Autodesk Fusion 360 part; units mm, degrees
note: some values were not read from the file. Chosen so that the rebuilt part matches the saved one: which bodies a step acts on; that a step has no effect.
(part 2 of 2)
sketch "Sketch27" plane through (0, 1.55, 0) normal (0, 1, 0) x (-1, 0, 0)
  circle A0 centre (-8.4, -28.1) radius 0.5
  circle A1 centre (-13.4, -28.1) radius 0.5
  circle A2 centre (-18.4, -28.1) radius 0.5
  line L0 (-19.48, -2.52) -> (-19.98, -2.52)
  line L1 (-19.98, -2.52) -> (-19.98, -2.02)
  line L2 (-19.98, -2.02) -> (-19.48, -2.02)
  line L3 (-19.48, -2.02) -> (-19.48, -2.52)
  line L4 (-16.94, -2.52) -> (-17.44, -2.52)
  line L5 (-17.44, -2.52) -> (-17.44, -2.02)
  line L6 (-17.44, -2.02) -> (-16.94, -2.02)
  line L7 (-16.94, -2.02) -> (-16.94, -2.52)
  line L8 (-14.4, -2.52) -> (-14.9, -2.52)
  line L9 (-14.9, -2.52) -> (-14.9, -2.02)
  line L10 (-14.9, -2.02) -> (-14.4, -2.02)
  line L11 (-14.4, -2.02) -> (-14.4, -2.52)
  circle A3 centre (-2.275, -2.375) radius 1.475
  circle A4 centre (-23.725, -2.375) radius 1.475
  circle A5 centre (-23.725, -31.325) radius 1.475
  circle A6 centre (-2.275, -31.325) radius 1.475
  line L12 (0, -33.5) -> (0, 0)
  line L13 (0, 0) -> (-26, 0)
  line L14 (-26, 0) -> (-26, -33.5)
  line L15 (-26, -33.5) -> (0, -33.5)
  circle A7 centre (-2.275, -31.325) radius 1.525
  circle A8 centre (-2.275, -31.325) radius 1.625
  line L16 (-13, -33.5) -> (-13, -31.8167) construction
  circle A9 centre (-23.725, -31.325) radius 1.475
  circle A10 centre (-23.725, -31.325) radius 1.625
  circle A11 centre (-2.275, -2.375) radius 1.525
  circle A12 centre (-2.275, -2.375) radius 1.625
  circle A13 centre (-23.725, -2.375) radius 1.625
  circle A14 centre (-23.725, -2.375) radius 1.525
  line L17 (-13.33, -3.59) -> (-21.05, -3.59)
  line L18 (-21.05, -3.59) -> (-21.05, -0.95)
  line L19 (-21.05, -0.95) -> (-13.33, -0.95)
  line L20 (-13.33, -0.95) -> (-13.33, -3.59)
  line L21 (-13.38, -3.032) -> (-13.38, -1.508)
  line L22 (-15.412, -3.54) -> (-13.888, -3.54)
  line L23 (-18.968, -1) -> (-20.492, -1)
  line L24 (-21, -1.508) -> (-21, -3.032)
  line L25 (-21.15, -0.85) -> (-13.23, -0.85)
  line L26 (-13.23, -0.85) -> (-13.23, -3.69)
  line L27 (-13.23, -3.69) -> (-21.15, -3.69)
  line L28 (-21.15, -3.69) -> (-21.15, -0.85)
  line L29 (-12.6, -0.3) -> (-21.5, -0.3) construction
  line L30 (-7.1042, -0.3) -> (-11.1042, -0.3) construction
  line L31 (-2.45, -19.55) -> (-4.55, -19.55)
  line L32 (-4.55, -19.55) -> (-4.55, -15.05)
  line L33 (-4.55, -15.05) -> (-2.45, -15.05)
  line L34 (-2.45, -15.05) -> (-2.45, -19.55)
  line L35 (-2.5, -19.3) -> (-2.5, -15.3)
  line L36 (-4, -19.5) -> (-3, -19.5)
  line L37 (-4, -15.1) -> (-3, -15.1)
  line L38 (-4.5, -15.3) -> (-4.5, -19.3)
  line L39 (-4.65, -19.65) -> (-4.65, -14.95)
  line L40 (-4.65, -14.95) -> (-2.35, -14.95)
  line L41 (-2.35, -14.95) -> (-2.35, -19.65)
  line L42 (-2.35, -19.65) -> (-4.65, -19.65)
  line L43 (-2.35, -19.65) -> (0, -19.65) construction
  line L44 (-2.45, -11.85) -> (-4.55, -11.85)
  line L45 (-4.55, -11.85) -> (-4.55, -10.75)
  line L46 (-4.55, -10.75) -> (-2.45, -10.75)
  line L47 (-2.45, -10.75) -> (-2.45, -11.85)
  line L48 (-4.5, -11.8) -> (-2.5, -11.8)
  line L49 (-2.5, -10.8) -> (-4.5, -10.8)
  line L50 (-2.5, -11.8) -> (-2.5, -10.8)
  line L51 (-4.5, -10.8) -> (-4.5, -11.8)
  line L52 (-2.35, -10.65) -> (-2.35, -11.95)
  line L53 (-2.35, -11.95) -> (-4.65, -11.95)
  line L54 (-4.65, -11.95) -> (-4.65, -10.65)
  line L55 (-4.65, -10.65) -> (-2.35, -10.65)
  line L56 (-2.25, -9.1) -> (-3.35, -9.1)
  line L57 (-3.35, -9.1) -> (-3.35, -7.4)
  line L58 (-3.35, -7.4) -> (-2.25, -7.4)
  line L59 (-2.25, -7.4) -> (-2.25, -9.1)
  line L60 (-2.3, -9.05) -> (-3.3, -9.05)
  line L61 (-2.3, -9) -> (-2.3, -7.5)
  line L62 (-3.3, -7.5) -> (-3.3, -9)
  line L63 (-2.3, -7.45) -> (-3.3, -7.45)
  line L64 (-2.15, -7.3) -> (-2.15, -9.2)
  line L65 (-2.15, -9.2) -> (-3.45, -9.2)
  line L66 (-3.45, -9.2) -> (-3.45, -7.3)
  line L67 (-3.45, -7.3) -> (-2.15, -7.3)
  line L68 (-7.7, -2.55) -> (-10.4, -2.55)
  line L69 (-10.4, -2.55) -> (-10.4, -1.45)
  line L70 (-10.4, -1.45) -> (-7.7, -1.45)
  line L71 (-7.7, -1.45) -> (-7.7, -2.55)
  line L72 (-7.75, -1.5) -> (-7.75, -2.5)
  line L73 (-10.3, -2.5) -> (-7.8, -2.5)
  line L74 (-7.8, -1.5) -> (-10.3, -1.5)
  line L75 (-10.35, -2.5) -> (-10.35, -1.5)
  line L76 (-7.6, -1.35) -> (-7.6, -2.65)
  line L77 (-7.6, -2.65) -> (-10.5, -2.65)
  line L78 (-10.5, -2.65) -> (-10.5, -1.35)
  line L79 (-10.5, -1.35) -> (-7.6, -1.35)
  line L80 (-5.85, -23.55) -> (-21.05, -23.55)
  line L81 (-21.05, -23.55) -> (-21.05, -4.45)
  line L82 (-21.05, -4.45) -> (-5.85, -4.45)
  line L83 (-5.85, -4.45) -> (-5.85, -23.55)
  line L84 (-21, -4.5) -> (-21, -23.5)
  line L85 (-15.1, -4.5) -> (-21, -4.5)
  line L86 (-5.9, -23.5) -> (-5.9, -4.5)
  line L87 (-21, -23.5) -> (-5.9, -23.5)
  line L88 (-5.75, -4.35) -> (-5.75, -23.65)
  line L89 (-5.75, -23.65) -> (-21.15, -23.65)
  line L90 (-21.15, -23.65) -> (-21.15, -4.35)
  line L91 (-21.15, -4.35) -> (-5.75, -4.35)
  line L92 (-5.85, -31.25) -> (-20.95, -31.25)
  line L93 (-20.95, -31.25) -> (-20.95, -23.55)
  line L94 (-20.95, -23.55) -> (-5.85, -23.55)
  line L95 (-5.85, -23.55) -> (-5.85, -31.25)
  line L96 (-5.9, -23.6) -> (-20.9, -23.6)
  line L97 (-5.9, -30.4) -> (-5.9, -25.4)
  line L98 (-5.9, -31.2) -> (-20.9, -31.2)
  line L99 (-20.9, -31.2) -> (-20.9, -30.4)
  line L100 (-21.05, -23.45) -> (-5.75, -23.45)
  line L101 (-5.75, -23.45) -> (-5.75, -31.35)
  line L102 (-5.75, -31.35) -> (-21.05, -31.35)
  line L103 (-21.05, -31.35) -> (-21.05, -23.45)
  line L104 (-5.75, -31.55) -> (-21.05, -31.55) construction
  line L105 (-2.35, -11.95) -> (0, -11.95) construction
  dimension "d175" = 3.05
  dimension "d176" = 0.1
  dimension "d228" = 3.05
  dimension "d229" = 0.1
  dimension "d230" = 0.05
  dimension "d231" = 0.05
  dimension "d232" = 0.05
  dimension "d233" = 0.05
  dimension "d234" = -0.1
  dimension "d235" = 0.3
  dimension "d236" = 0.3
  dimension "d237" = 4
  dimension "d238" = 0.05
  dimension "d239" = 0.05
  dimension "d240" = 0.05
  dimension "d241" = 0.05
  dimension "d242" = -0.1
  dimension "d243" = 0.05
  dimension "d244" = 0.05
  dimension "d245" = 0.05
  dimension "d246" = 0.05
  dimension "d247" = -0.1
  dimension "d248" = 0.05
  dimension "d249" = 0.05
  dimension "d250" = 0.05
  dimension "d251" = 0.05
  dimension "d252" = -0.1
  dimension "d253" = 0.05
  dimension "d254" = 0.05
  dimension "d255" = 0.05
  dimension "d256" = 0.05
  dimension "d257" = -0.1
  dimension "d258" = 0.05
  dimension "d259" = 0.05
  dimension "d260" = 0.05
  dimension "d261" = 0.05
  dimension "d262" = -0.1
  dimension "d263" = 0.05
  dimension "d264" = 0.05
  dimension "d265" = 0.05
  dimension "d266" = 0.05
  dimension "d267" = -0.1
  dimension "d268" = 15.3
  dimension "d269" = 0.2
  constraint concentric A6 A7
  constraint midpoint L15 L16.start
  constraint perpendicular L15 L16
  constraint symmetric A6 L16 A9
  constraint symmetric A8 L16 A10
  constraint concentric A3 A11
  constraint symmetric L16 A11 A14
  constraint symmetric L16 A12 A13
  constraint horizontal L17
  constraint vertical L18
  constraint horizontal L19
  constraint vertical L20
  constraint perpendicular L11 L29
  constraint parallel L13 L30
  constraint horizontal L31
  constraint vertical L32
  constraint horizontal L33
  constraint vertical L34
  constraint coincident L12 L43.end
  constraint perpendicular L12 L43
  constraint horizontal L44
  constraint vertical L45
  constraint horizontal L46
  constraint vertical L47
  constraint horizontal L56
  constraint vertical L57
  constraint horizontal L58
  constraint vertical L59
  constraint horizontal L68
  constraint vertical L69
  constraint horizontal L70
  constraint vertical L71
  constraint horizontal L80
  constraint vertical L81
  constraint horizontal L82
  constraint vertical L83
  constraint horizontal L92
  constraint vertical L93
  constraint horizontal L94
  constraint vertical L95
  constraint perpendicular L103 L104
  constraint coincident L12 L105.end
  constraint perpendicular L12 L105
  measures "d175" diameter of A7
  measures "d228" diameter of A11
  measures "d230" distance of L20 L21
  measures "d231" distance of L17 L22
  measures "d232" distance of L19 L23
  measures "d233" distance of L18 L24
  measures "d235" distance of L13 L29
  measures "d236" distance of L13 L30
  measures "d237" distance of L30.start L30.end
  measures "d238" distance of L34 L35
  measures "d239" distance of L31 L36
  measures "d240" distance of L33 L37
  measures "d241" distance of L32 L38
  measures "d243" distance of L44 L48
  measures "d244" distance of L46 L49
  measures "d245" distance of L47 L50
  measures "d246" distance of L45 L51
  measures "d248" distance of L56 L60
  measures "d249" distance of L59 L61
  measures "d250" distance of L57 L62
  measures "d251" distance of L58 L63
  measures "d253" distance of L71 L72
  measures "d254" distance of L68 L73
  measures "d255" distance of L70 L74
  measures "d256" distance of L69 L75
  measures "d258" distance of L81 L84
  measures "d259" distance of L82 L85
  measures "d260" distance of L83 L86
  measures "d261" distance of L80 L87
  measures "d263" distance of L94 L96
  measures "d264" distance of L95 L97
  measures "d265" distance of L92 L98
  measures "d266" distance of L93 L99
  measures "d268" distance of L104.start L104.end
  measures "d269" distance of L102 L104
extrude "Extrude21" [no effect]
equation "d29 = ( 2.54 * 3 ) * 1 mm"
equation "d36 = ( 2.54 / 5 ) * 1 mm"
equation "d37 = ( 2.54 / 2 ) * 1 mm"
equation "d66 = ( -2.54 / 2 ) * 1 mm"
equation "d98 = -( 7.6 mm - 1.8 mm )"
equation "d130 = ( ( 3 / 5 ) * 2.8 ) * 1 mm"
equation "d139 = ( 0.75 / 2 ) * 1 mm"
named bodies: "Board", "Relay", "Pin Base", "Ground", "5V Pin", "Sig Pin", "Termial Block", "NO", "COM", "NC", "LED"
